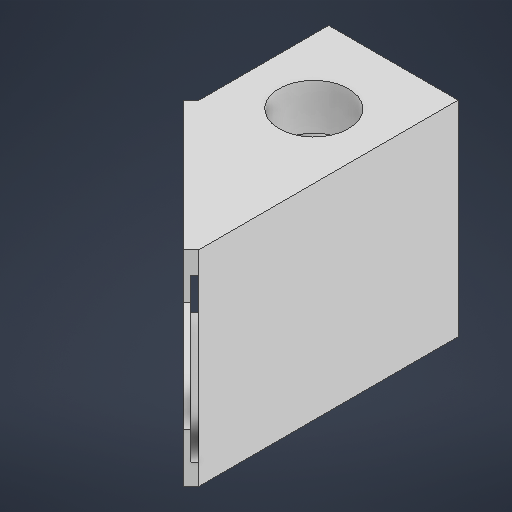
# Autodesk Inventor part: Camera Holder V2 BP Height and 45 Deg
Saved by Autodesk Inventor 2026 (Build 300175000, 175)
## iProperties
Created: 2026-01-21
Part Number: Camera Holder V2 BP Height and 45 Deg
Material: Generic
Document SubType Name: Modeling
Designer: FiolkaLab
Density: 1 g/cm^3
Appearance: Default
Author: FiolkaLab
Autodesk Inventor part; units mm, degrees
ref_plane "YZ Plane" through (0, 0, 0) normal (1, 0, 0) x (0, 1, 0)
ref_plane "XZ Plane" through (0, 0, 0) normal (0, 1, 0) x (-1, 0, 0)
ref_plane "XY Plane" through (0, 0, 0) normal (0, 0, 1) x (1, 0, 0)
sketch "Sketch1" plane through (0, 0, 0) normal (0, 0, 1) x (1, 0, 0)
  line L0 (9, 14.25) -> (-9, 14.25)
  line L1 (-9, 14.25) -> (-9, -14.25)
  line L2 (-9, -14.25) -> (9, -14.25)
  line L3 (9, -14.25) -> (9, 14.25)
  line L4 (9, 14.25) -> (-9, -14.25) construction
  line L5 (-9, 14.25) -> (9, -14.25) construction
  point P0 (0, 0)
  dimension "d0" = 28.5
  dimension "d1" = 18
  constraints: 12 end point, 2 midpoint, 2 parallel, 1 horizontal, 1 perpendicular
  measures "d0" distance of L2.end L0.start
  measures "d1" distance of L1.end L2.end
extrude "Extrusion1" add sketch "Sketch1" against normal blind 25.4
sketch "Sketch3" plane through (0, 0, -25.4) normal (0, 0, -1) x (-1, 0, 0)
  line L0 (-7.625, 7.875) -> (7.625, 7.875)
  line L1 (7.625, 7.875) -> (7.625, -7.375)
  line L2 (7.625, -7.375) -> (-7.625, -7.375)
  line L3 (-7.625, -7.375) -> (-7.625, 7.875)
  line L4 (-9, -14.25) -> (9, -14.25) projected
  line L5 (9, -14.25) -> (9, 14.25) projected
  line L6 (9, 14.25) -> (-9, 14.25) projected
  point P0 (0, 0)
  dimension "d7" = 15.25
  dimension "d8" = 15.25
  dimension "d10" = 1.375
  dimension "d186" = 6.375
  constraints: 8 end point, 2 parallel, 1 horizontal, 1 perpendicular
  measures "d7" distance of L0.end L1.end
  measures "d8" distance of L0.start L0.end
  measures "d10" distance between parallel lines of L5 L1
  measures "d186" distance between parallel lines of L6 L0
extrude "Extrusion2" cut sketch "Sketch3" against normal blind 23.4
sketch "Sketch4" plane through (0, 0, 0) normal (0, 0, 1) x (1, 0, 0)
  line L0 (-7.625, 7.875) -> (-7.625, -7.375) projected
  line L1 (-7.625, -7.375) -> (7.625, -7.375) projected
  line L2 (7.625, -7.375) -> (7.625, 7.875) projected
  line L3 (7.625, 7.875) -> (-7.625, 7.875) projected
  line L4 (-9, -14.25) -> (-9, 14.25) projected
  line L5 (-9, 14.25) -> (9, 14.25) projected
  line L6 (9, 14.25) -> (9, -14.25) projected
  line L7 (9, -14.25) -> (-9, -14.25) projected
  line L8 (7.625, -7.375) -> (4.625, -7.375)
  line L9 (7.625, -7.375) -> (7.625, -4.375)
  line L10 (7.625, -4.375) -> (6.25, -4.375)
  line L11 (4.625, -7.375) -> (4.625, -6)
  line L12 (4.625, -6) -> (6.25, -4.375)
  line L13 (7.625, 7.875) -> (-7.625, 7.875) projected
  line L14 (-7.625, 7.875) -> (-4.625, 7.875)
  line L15 (-4.625, 7.875) -> (-4.625, 6.5)
  line L16 (-7.625, 7.875) -> (-7.625, -7.375) projected
  line L17 (-7.625, 7.875) -> (-7.625, 4.875)
  line L18 (-7.625, 4.875) -> (-6.25, 4.875)
  line L19 (-6.25, 4.875) -> (-4.625, 6.5)
  point P0 (0, 0)
  dimension "d21" = 3
  dimension "d22" = 3
  dimension "d23" = 1.375
  dimension "d24" = 1.375
  dimension "d60" = 3
  dimension "d61" = 1.375
  dimension "d62" = 3
  dimension "d63" = 1.375
  constraints: 20 end point, 4 point on line, 2 vertical, 1 horizontal, 1 perpendicular
  measures "d21" distance of L1.end L8.end
  measures "d22" distance of L1.end L9.end
  measures "d23" distance of L9.end L10.end
  measures "d24" distance of L8.end L11.end
  measures "d60" distance of L0.start L14.end
  measures "d61" distance of L14.end L15.end
  measures "d62" distance of L0.start L17.end
  measures "d63" distance of L17.end L18.end
sketch "Sketch6" plane through (-7.625, -7.375, -25.4) normal (0, 1, 0) x (1, 0, 0)
  line L0 (0, -23.4) -> (15.25, -23.4) projected
  point P0 (7.625, -25.4)
  point P1 (7.7785, -18.15)
  dimension "d20" = 5.25
  measures "d20" distance from line of L0 point (7.779, -18.15)
hole "Hole1" [suppressed]
sketch "Sketch7" plane through (0, 0, 0) normal (0, 0, 1) x (1, 0, 0)
  line L0 (-7.625, -7.375) -> (7.625, -7.375) projected
  line L1 (4.6166, -7.375) -> (4.6166, -6.0121)
  line L2 (4.6166, -6.0121) -> (6.2367, -4.3791)
  line L3 (6.2367, -4.3791) -> (7.625, -4.3791)
  line L4 (7.625, -4.3791) -> (7.625, 7.8472)
  line L5 (7.625, 7.875) -> (-7.625, 7.875) projected
  line L6 (7.625, 7.8472) -> (-7.625, 7.875)
  line L7 (-7.625, 7.875) -> (-7.625, -7.375)
  line L8 (-7.625, -7.375) -> (4.6166, -7.375)
  point P0 (0, 0)
  constraints: 14 end point, 3 perpendicular, 1 parallel, 1 point on line, 1 vertical
extrude "Extrusion3" cut sketch "Sketch4" against normal through all contours L3 L15 L19 L18 L0 | L18 L19 L15 L3 L2 L10 L12 L11 L1 L0
sketch "Sketch8" plane through (0, 0, 0) normal (0, 0, 1) x (1, 0, 0)
  circle A0 centre (6.25, -6) radius 1.05
  line L0 (4.625, -6) -> (4.625, -7.375) projected
  line L1 (7.625, -4.375) -> (6.25, -4.375) projected
  point P0 (0, 0)
  dimension "d27" = 2.1
  dimension "d28" = 1.625
  dimension "d29" = 1.625
  constraints: 1 centre point
  measures "d27" diameter of A0
  measures "d28" distance from line of L0 A0.centre
  measures "d29" distance from line of L1 A0.centre
extrude "Extrusion4" cut sketch "Sketch8" against normal blind 25.4
sketch "Sketch9" plane through (4.625, -6, -2) normal (-0.7071068, 0.7071068, 0) x (-0.7071068, -0.7071068, 0)
  line L0 (0, 0) -> (-2.2981, 0) projected
  line L1 (0, 2) -> (0, 0) projected
  line L2 (-2.2981, 2) -> (0, 2) projected
  line L3 (-2.2981, 2) -> (-2.2981, 0) projected
  point P0 (-0.9723, 2)
extrude "Extrusion5" add sketch "Sketch9" along normal blind 0.175
sketch "Sketch10" plane through (0, 0, -25.4) normal (0, 0, -1) x (-1, 0, 0)
  line L0 (-7.625, -7.375) -> (-7.625, 7.875) projected
  line L1 (-9, 14.25) -> (-9, -14.25) projected
  circle A0 centre (-7.225, -6.925) radius 0.8
  line L2 (7.625, -7.375) -> (-7.625, -7.375) projected
  point P0 (0, 0)
  dimension "d41" = 1.6
  dimension "d42" = 1.775
  dimension "d46" = 1.25
  constraints: 1 centre point
  measures "d41" diameter of A0
  measures "d42" distance from line of L1 A0.centre
extrude "Extrusion6" cut sketch "Sketch10" against normal up to surface (23.4 mm away)
pattern_linear "Rectangular Pattern1" count 2 spacing 14.45 along (-1, 0, 0) count 2 spacing 14.45 along (0, 1, 0) of "Extrusion6" first direction both ways yes
sketch "Sketch15" plane through (0, 0, 0) normal (0, 0, 1) x (1, 0, 0)
  line L0 (-7.625, 7.875) -> (7.625, 7.875) projected
  line L1 (-7.625, 7.875) -> (-4.625, 7.875)
  line L2 (-7.625, -7.375) -> (-7.625, 7.875) projected
  line L3 (-7.625, 7.875) -> (-7.625, 4.875)
  line L4 (-7.625, 4.875) -> (-6.25, 4.875)
  line L5 (-4.625, 7.875) -> (-4.625, 6.5)
  line L6 (-4.625, 6.5) -> (-6.25, 4.875)
  point P0 (0, 0)
  dimension "d64" = 3
  dimension "d65" = 3
  dimension "d66" = 1.375
  dimension "d67" = 1.375
  constraints: 10 end point, 2 perpendicular, 2 point on line
  measures "d64" distance of L0.start L1.end
  measures "d65" distance of L0.start L3.end
  measures "d66" distance of L3.end L4.end
  measures "d67" distance of L1.end L5.end
extrude "Extrusion9" add sketch "Sketch15" against normal blind 2
sketch "Sketch16" plane through (0, 0, 0) normal (0, 0, 1) x (1, 0, 0)
  circle A0 centre (-6.25, 6.5) radius 1.05
  line L0 (-7.625, 4.875) -> (-6.25, 4.875) projected
  line L1 (-4.625, 6.5) -> (-4.625, 7.875) projected
  point P0 (0, 0)
  dimension "d70" = 2.1
  dimension "d71" = 1.625
  dimension "d72" = 1.625
  constraints: 1 centre point
  measures "d70" diameter of A0
  measures "d71" distance from line of L0 A0.centre
  measures "d72" distance from line of L1 A0.centre
extrude "Extrusion10" cut sketch "Sketch16" against normal blind 2
sketch "Sketch11" plane through (-9, 14.25, 0) normal (0, 1, 0) x (1, 0, 0)
  circle A0 centre (9.1535, 7.25) radius 4.8 projected
  point P0 (9, 0)
extrude "Extrusion7" [suppressed]
chamfer "Chamfer1" [suppressed]
sketch "Sketch14" plane through (-7.625, -13.2465, 0) normal (-0.7660444, 0, 0.6427876) x (0.6427876, 0, 0.7660444)
  line L0 (-2.1391, 0) -> (0, 0) projected
  line L1 (0, 0) -> (0, 4.868) projected
  line L2 (0, 26.493) -> (-2.1391, 26.493) projected
  line L3 (-2.1391, 26.493) -> (-2.1391, 0) projected
  line L4 (0, 4.868) -> (0, 17.118) projected
  line L5 (0, 17.118) -> (0, 26.493) projected
  point P0 (4.9013, 13.2465)
extrude "Extrusion8" [suppressed]
chamfer "Chamfer2" [suppressed]
sketch "Sketch17" plane through (-6.25, 4.875, 0) normal (0.7071068, -0.7071068, 0) x (-0.7071068, -0.7071068, 0)
  line L0 (0, 0) -> (-2.2981, 0) projected
  line L1 (0, 0) -> (0, 2) projected
  line L2 (-2.2981, 2) -> (0, 2) projected
  line L3 (-2.2981, 0) -> (-2.2981, 2) projected
  point P0 (-0.9723, 0)
extrude "Extrusion11" add sketch "Sketch17" along normal blind 0.175
sketch "Sketch18" plane through (7.625, -13.2465, 0) normal (0.8660254, 0, 0.5) x (0.5, 0, -0.8660254)
  line L0 (2.75, 26.493) -> (0, 26.493) projected
  line L1 (0, 26.493) -> (0, 20.118) projected
  line L2 (0, 0) -> (2.75, 0) projected
  line L3 (2.75, 0) -> (2.75, 26.493) projected
  line L4 (0, 20.118) -> (0, 7.868) projected
  line L5 (0, 7.868) -> (0, 0) projected
  point P0 (-3.8125, 13.2465)
extrude "Extrusion12" [suppressed]
sketch "Sketch26" plane through (-9, 14.25, -25.4) normal (0, 1, 0) x (1, 0, 0)
  line L0 (1.375, -25.4) -> (-2.0891, -27.4) projected
  line L1 (21.4641, -25.0184) -> (20.0891, -27.4) projected
  line L2 (-2.0891, -27.4) -> (20.0891, -27.4)
  line L3 (20.0891, -27.4) -> (16.625, -25.4)
  line L4 (18, -25.4) -> (0, -25.4) projected
  line L5 (16.625, -25.4) -> (1.375, -25.4)
  line L6 (1.375, -25.4) -> (-2.0891, -27.4)
  point P0 (9, -25.4)
  point P1 (16.625, -25.4)
  point P2 (16.625, -25.4)
  constraints: 8 end point, 1 horizontal, 1 parallel, 1 perpendicular
extrude "Extrusion19" [suppressed]
sketch "Sketch27" plane through (4.625, -7.375, 0) normal (0, 1, 0) x (1, 0, 0)
  line L0 (-9.25, 0) -> (-9.25, 2) projected
  line L1 (-9.25, 2) -> (-11.1306, 2) projected
  line L2 (-11.1306, 2) -> (-11.1306, 25.4) projected
  line L3 (1.8806, 25.4) -> (-11.1306, 25.4) projected
  line L4 (1.8806, 25.4) -> (1.8806, 2) projected
  line L5 (1.8806, 2) -> (3, 2) projected
  line L6 (3, 2) -> (3, 0) projected
  line L7 (-9.25, 0) -> (3, 0) projected
  line L8 (0, 0) -> (-12.25, 0) projected
  line L9 (-12.25, 0) -> (3, 0)
  point P0 (-4.625, 0)
  constraints: 2 end point, 1 collinear
extrude "Extrusion20" add sketch "Sketch27" against normal up to surface (6.875 mm away)
sketch "Sketch29" plane through (-11.0891, 13.2465, 2) normal (0, 0, 1) x (1, 0, 0)
  line L0 (22.1782, 0) -> (22.1782, -6.375) projected
  line L1 (0, -6.375) -> (0, 0) projected
  line L2 (22.1782, -1) -> (0, -1)
  line L3 (0, -1) -> (0, 0)
  line L4 (0, 0) -> (22.1782, 0)
  line L5 (22.1782, 0) -> (22.1782, -1)
  point P0 (11.0891, -13.2465)
  point P1 (0, -1)
  dimension "d102" = 1
  constraints: 8 end point, 2 parallel, 1 horizontal, 1 perpendicular, 1 point on line
  measures "d102" distance between parallel lines of L4 L2
extrude "Extrusion21" [suppressed]
sketch "Sketch30" plane through (-11.0891, -8.3785, 2) normal (0, 0, 1) x (1, 0, 0)
  line L0 (22.1782, 0) -> (22.1782, -4.868) projected
  line L1 (0, -4.868) -> (0, 0) projected
  line L2 (22.1782, -2.868) -> (0, -2.868)
  line L3 (0, -2.868) -> (0, -4.868)
  line L4 (0, -4.868) -> (22.1782, -4.868)
  line L5 (22.1782, -4.868) -> (22.1782, -2.868)
  point P0 (11.0891, 8.3785)
  point P1 (0, -2.868)
  dimension "d105" = 2
  constraints: 8 end point, 2 parallel, 1 horizontal, 1 perpendicular, 1 point on line
  measures "d105" distance between parallel lines of L4 L2
extrude "Extrusion22" [suppressed]
sketch "Sketch31" plane through (-11.0891, -11.2465, 2) normal (0, 1, 0) x (1, 0, 0)
  line L0 (22.1782, 0) -> (22.1782, -0.75) projected
  line L1 (0, -0.75) -> (22.1782, -0.75)
  line L2 (22.1782, -0.75) -> (22.1782, -0.5)
  line L3 (22.1782, -0.5) -> (0, -0.5)
  line L4 (0, -0.5) -> (0, -0.75)
  point P0 (11.0891, 2)
  dimension "d108" = 0.25
  constraints: 8 end point, 2 parallel, 1 horizontal, 1 perpendicular, 1 point on line
  measures "d108" distance between parallel lines of L1 L3
extrude "Extrusion23" [suppressed]
sketch "Sketch32" plane through (-11.0891, 12.2465, 2) normal (0, -1, 0) x (1, 0, 0)
  line L0 (21.8032, 0.75) -> (21.8032, 0.5) projected
  line L1 (21.8032, 0.5) -> (0, 0.5) projected
  line L2 (0, 0.5) -> (0, 0.75) projected
  line L3 (0, 0.75) -> (21.8032, 0.75) projected
  point P0 (11.0891, -2)
extrude "Extrusion24" [suppressed]
fillet "Fillet3" radius 1.27 1 edges at (6.1263, -4.2513, -1)
fillet "Fillet4" radius 1.27 1 edges at (4.5013, -5.8763, -1)
fillet "Fillet5" radius 1.27 2 edges at (-4.5013, 6.3763, -1) (-6.1263, 4.7513, -1)
chamfer "Chamfer7" distance 0.5 angle 45 8 edges at (7.625, -6.2322, -13.7) (6.5636, -7.375, -13.7) (7.625, 6.8322, -13.7) (6.5056, 7.875, -13.7) (-6.5636, -7.375, -13.7) (-7.625, -6.2322, -13.7) (-7.625, 6.8322, -13.7) (-6.5056, 7.875, -13.7)
chamfer "Chamfer8" [suppressed]
fillet "Fillet6" [suppressed]
chamfer "Chamfer10" [suppressed]
fillet "Fillet9" [suppressed]
fillet "Fillet10" [suppressed]
chamfer "Chamfer11" [suppressed]
fillet "Fillet11" [suppressed]
sketch "Sketch42" plane through (0, 0, 0) normal (0, 0, 1) x (1, 0, 0)
  line L0 (-9, -14.25) -> (9, -14.25) projected
  line L1 (9, 14.25) -> (-9, 14.25) projected
  line L2 (-9, -14.25) -> (9, -14.25)
  line L3 (9, -14.25) -> (9, 14.25)
  line L4 (9, 14.25) -> (-9, 14.25)
  line L5 (-9, 14.25) -> (-9, -14.25)
  line L6 (-7.625, -7.375) -> (-7.625, -5.7322) projected
  line L7 (7.625, 7.875) -> (7.625, -4.375) projected
  line L8 (-7.625, -7.375) -> (7.625, -7.375)
  line L9 (7.625, -7.375) -> (7.625, 7.875)
  line L10 (7.625, 7.875) -> (-7.625, 7.875)
  line L11 (-7.625, 7.875) -> (-7.625, -7.375)
  point P0 (0, 0)
  point P1 (7.625, -4.375)
  constraints: 16 end point, 4 parallel, 2 horizontal, 2 perpendicular
extrude "Extrusion28" [suppressed]
sketch "Sketch43" plane through (-9, 14.25, -25.4) normal (0, 1, 0) x (1, 0, 0)
  line L0 (0, -45.213) -> (18, -45.213)
  line L1 (18, -45.213) -> (0, -27.213)
  line L2 (0, -27.213) -> (0, -45.213)
  point P0 (9, -25.4)
  dimension "d154" = 45
  constraints: 6 end point, 1 perpendicular
  measures "d154" angle of L1 L0
extrude "Extrusion29" [suppressed]
sketch "Sketch45" plane through (9, -14.25, 19.813) normal (-0.7071068, 0, 0.7071068) x (0.7071068, 0, 0.7071068)
  line L0 (-25.4558, 28.5) -> (2.5472, 28.5)
  line L1 (2.5472, 28.5) -> (2.5472, 27.5094)
  line L2 (2.5472, 27.5094) -> (-25.4558, 27.5094)
  line L3 (-25.4558, 27.5094) -> (-25.4558, 28.5)
  line L4 (-25.4558, 0) -> (2.5472, 0)
  line L5 (2.5472, 0) -> (2.5472, 3.7596)
  line L6 (2.5472, 3.7596) -> (-25.4558, 3.7596)
  line L7 (-25.4558, 3.7596) -> (-25.4558, 0)
  point P0 (-20.3739, 14.25)
  dimension "d166" = 0.9906
  dimension "d167" = 3.7596
  constraints: 16 end point, 4 parallel, 2 horizontal, 2 perpendicular
  measures "d166" distance between parallel lines of L0 L2
  measures "d167" distance between parallel lines of L6 L4
extrude "Extrusion30" [suppressed]
sketch "Sketch47" plane through (9, -10.4904, 19.813) normal (0, 1, 0) x (0.7071068, 0, -0.7071068)
  line L0 (-2, -2.5472) -> (-2, 25.4558) projected
  line L1 (0, -2.5472) -> (-2, -2.5472) projected
  line L2 (-2, 25.4558) -> (0.622, 25.4558)
  line L3 (0.622, 25.4558) -> (0.622, -2.5472)
  line L4 (0.622, -2.5472) -> (-2, -2.5472)
  line L5 (-2, -2.5472) -> (-2, 25.4558)
  point P0 (7.6459, 20.3739)
  point P1 (0, 0)
  dimension "d173" = 2.622
  constraints: 8 end point, 2 parallel, 1 horizontal, 1 perpendicular, 2 other
  measures "d173" distance of L3.end L4.end
extrude "Extrusion32" [suppressed]
sketch "Sketch48" plane through (-9, 13.2594, 1.813) normal (0, -1, 0) x (0.7071068, 0, -0.7071068)
  line L0 (-2, 0) -> (-2, 28.003) projected
  line L1 (-2, 28.003) -> (0.622, 28.003) projected
  line L2 (0.622, 28.003) -> (0.622, 24.8338) projected
  line L3 (0, 0) -> (-2, 0) projected
  line L4 (0, 0) -> (0, 25.4558) projected
  line L5 (0, 25.4558) -> (0.622, 24.8338) projected
  point P0 (7.6459, 5.082)
extrude "Extrusion33" [suppressed]
chamfer "Chamfer12" [suppressed]
chamfer "Chamfer13" [suppressed]
sketch "Sketch51" plane through (-8.365, -14.25, -24.765) normal (0, -1, 0) x (1, 0, 0)
  line L0 (17.365, -0.635) -> (-0.635, -0.635) projected
  line L1 (-0.635, 24.765) -> (17.365, 24.765) projected
  line L2 (-0.635, 24.765) -> (-0.635, -0.635) projected
  line L3 (17.365, 24.765) -> (17.365, -0.635) projected
  point P0 (8.365, 24.765)
extrude "Extrusion34" [suppressed]
sketch "Sketch52" plane through (-9, 14.25, 0) normal (0, 1, 0) x (1, 0, 0)
  line L0 (0, 0) -> (0, -18)
  line L1 (0, -18) -> (18, -18)
  line L2 (18, -18) -> (0, 0)
  point P0 (9, 0)
  dimension "d189" = 45
  constraints: 6 end point, 1 perpendicular, 1 vertical
  measures "d189" angle of L2 L1
sketch "Sketch54" plane through (0, 0, 0) normal (0, 0, 1) x (1, 0, 0)
  line L0 (-9, 14.25) -> (-9, -14.25) projected
  line L1 (9, -14.25) -> (9, 14.25) projected
  line L2 (-9, 7.875) -> (9, 7.875)
  line L3 (9, 7.875) -> (9, 14.25)
  line L4 (9, 14.25) -> (-9, 14.25)
  line L5 (-9, 14.25) -> (-9, 7.875)
  line L6 (-7.625, -7.375) -> (-7.625, -5.7322) projected
  line L7 (-9, 7.875) -> (-7.625, 7.875)
  line L8 (-7.625, 7.875) -> (-7.625, -7.375)
  line L9 (-7.625, -7.375) -> (-9, -7.375)
  line L10 (-9, -7.375) -> (-9, 7.875)
  line L11 (9, 7.875) -> (7.625, 7.875)
  line L12 (7.625, 7.875) -> (7.625, -7.375)
  line L13 (7.625, -7.375) -> (9, -7.375)
  line L14 (9, -7.375) -> (9, 7.875)
  line L15 (-9, -7.375) -> (9, -7.375)
  line L16 (9, -7.375) -> (9, -14.25)
  line L17 (9, -14.25) -> (-9, -14.25)
  line L18 (-9, -14.25) -> (-9, -7.375)
  point P0 (7.625, 7.875)
  point P1 (-9, -14.25)
  point P2 (9, -14.25)
  point P3 (7.625, -7.375)
  constraints: 32 end point, 8 parallel, 4 horizontal, 4 perpendicular, 3 point on line
extrude "Extrusion38" cut sketch "Sketch52" against normal through all
extrude "Extrusion40" add sketch "Sketch54" along normal blind 18 contours L4 L1 L2 L0 | L2 L8 L6 L9 L0 | L9 L15 L13 L1 L17 L0 | L1 L13 L12 L2
sketch "Sketch57" plane through (-9, 14.25, -25.4) normal (0, 1, 0) x (1, 0, 0)
  line L0 (18, 0) -> (18, -43.4) projected
  line L1 (0, -43.4) -> (18, -43.4)
  line L2 (18, -43.4) -> (0, -25.4)
  line L3 (0, -25.4) -> (0, -43.4)
  point P0 (9, -25.4)
  dimension "d203" = 45
  constraints: 6 end point, 1 perpendicular
  measures "d203" angle of L2 L1
extrude "Extrusion41" cut sketch "Sketch57" against normal through all
sketch "Sketch58" plane through (-7.625, 4.875, 0) normal (1, 0, 0) x (0, 0, -1)
  line L0 (-1.375, 3) -> (-1.375, -12.25) projected
  line L1 (0, 3) -> (-1.375, 3)
  line L2 (-1.375, 3) -> (-1.375, -12.25)
  line L3 (-1.375, -12.25) -> (0, -12.25)
  line L4 (0, -12.25) -> (0, 3)
  point P0 (0, -4.875)
  constraints: 8 end point, 2 parallel, 1 horizontal, 1 perpendicular
extrude "Extrusion42" cut sketch "Sketch58" against normal through all
sketch "Sketch59" plane through (9, -14.25, 18) normal (-0.7071068, 0, 0.7071068) x (0.7071068, 0, 0.7071068)
  line L0 (-25.4558, 28.5) -> (0, 28.5)
  line L1 (0, 28.5) -> (0, 25.452)
  line L2 (0, 25.452) -> (-25.4558, 25.452)
  line L3 (-25.4558, 25.452) -> (-25.4558, 28.5)
  line L4 (-25.4558, 0) -> (0, 0)
  line L5 (0, 0) -> (0, 2.952)
  line L6 (0, 2.952) -> (-25.4558, 2.952)
  line L7 (-25.4558, 2.952) -> (-25.4558, 0)
  point P0 (-19.0919, 14.25)
  dimension "d208" = 22.5
  dimension "d209" = 3.048
  constraints: 16 end point, 4 parallel, 2 horizontal, 2 perpendicular, 1 point on line
  measures "d208" distance between parallel lines of L6 L2
  measures "d209" distance between parallel lines of L0 L2
extrude "Extrusion43" add sketch "Sketch59" along normal blind 1.5
sketch "Sketch60" plane through (9, -11.298, 18) normal (0, 1, 0) x (0.7071068, 0, -0.7071068)
  line L0 (-1.5, 0) -> (-1.5, 25.4558) projected
  line L1 (-1.5, 25.4558) -> (-0.75, 25.4558)
  line L2 (-0.75, 25.4558) -> (-0.75, 0)
  line L3 (-0.75, 0) -> (-1.5, 0)
  line L4 (-1.5, 0) -> (-1.5, 25.4558)
  point P0 (6.364, 19.0919)
  point P1 (-1.5, 0)
  dimension "d213" = 0.75
  constraints: 8 end point, 2 parallel, 1 horizontal, 1 perpendicular
  measures "d213" distance between parallel lines of L0 L2
extrude "Extrusion44" add sketch "Sketch60" along normal up to surface (3.923 mm away)
sketch "Sketch61" plane through (-9, 11.202, 0) normal (0, -1, 0) x (0.7071068, 0, -0.7071068)
  line L0 (-1.5, 25.4558) -> (-0.75, 25.4558) projected
  line L1 (-0.75, 25.4558) -> (-0.75, 0) projected
  line L2 (-0.75, 0) -> (-1.5, 0) projected
  line L3 (-1.5, 0) -> (-1.5, 25.4558) projected
  point P0 (6.364, 6.364)
extrude "Extrusion45" add sketch "Sketch61" along normal up to surface (3.327 mm away)
sketch "Sketch62" plane through (0, 0, 0) normal (0, 0, 1) x (1, 0, 0)
  line L0 (-7.625, 4.875) -> (-9, 4.875)
  line L1 (-9, 4.875) -> (-9, -7.375)
  line L2 (-9, -7.375) -> (-7.625, -7.375)
  line L3 (-7.625, -7.375) -> (-7.625, 4.875)
  point P0 (0, 0)
  constraints: 8 end point, 2 parallel, 1 horizontal, 1 perpendicular
extrude "Extrusion46" cut sketch "Sketch62" against normal blind 1.5
sketch "Sketch63" plane through (0, 0, -25.4) normal (0, 0, -1) x (-1, 0, 0)
  line L0 (-9, -14.25) -> (9, -14.25) projected
  line L1 (9, -14.25) -> (9, 14.25) projected
  line L2 (9, 14.25) -> (-9, 14.25) projected
  line L3 (-9, 14.25) -> (-9, -14.25) projected
  line L4 (6.8539, 8.2337) -> (6.0056, 7.875) projected
  arc A0 (7.9582, 7.205) -> (6.8539, 8.2337) centre (7.225, 7.525) ccw projected
  line L5 (7.625, 6.3322) -> (7.9582, 7.205) projected
  line L6 (7.625, 6.3322) -> (7.625, -5.7322) projected
  line L7 (7.9582, -6.605) -> (7.625, -5.7322) projected
  arc A1 (6.9599, -7.6798) -> (7.9582, -6.605) centre (7.225, -6.925) ccw projected
  line L8 (6.0636, -7.375) -> (6.9599, -7.6798) projected
  line L9 (6.0636, -7.375) -> (-6.0636, -7.375) projected
  line L10 (-6.9599, -7.6798) -> (-6.0636, -7.375) projected
  arc A2 (-7.9582, -6.605) -> (-6.9599, -7.6798) centre (-7.225, -6.925) ccw projected
  line L11 (-7.625, -5.7322) -> (-7.9582, -6.605) projected
  line L12 (-7.625, -5.7322) -> (-7.625, 6.3322) projected
  line L13 (-7.9582, 7.205) -> (-7.625, 6.3322) projected
  arc A3 (-6.8539, 8.2337) -> (-7.9582, 7.205) centre (-7.225, 7.525) ccw projected
  line L14 (-6.0056, 7.875) -> (-6.8539, 8.2337) projected
  line L15 (-6.0056, 7.875) -> (6.0056, 7.875) projected
  point P0 (0, 0)
extrude "Extrusion47" cut sketch "Sketch63" against normal blind 7.31
sketch "Sketch64" plane through (4.625, -7.375, 0) normal (0, 1, 0) x (1, 0, 0)
  line L0 (0, 2) -> (1.4386, 2) projected
  point P0 (-4.625, 0)
  point P1 (-4.63, 7.025)
  point P2 (-12.25, 18.09)
  dimension "d229" = 5.025
  dimension "d230" = 7.62
  measures "d229" distance from line of L0 point (-4.63, 7.025)
  measures "d230" horizontal distance of point (-12.25, 18.09) point (-4.63, 7.025)
hole "Hole3" at (-0.005, -7.375, -7.025) direction (0, -1, 0) diameter 6.35 end through all counterbore diameter 9.652 counterbore depth 3.556
sketch "Sketch66" plane through (-9, 14.25, -18.09) normal (0, 1, 0) x (1, 0, 0)
  circle A0 centre (8.995, -11.065) radius 4.826 projected
  point P0 (9, -18.09)
extrude "Extrusion48" cut sketch "Sketch66" against normal up to surface (6.375 mm away)
body "Solid1"
